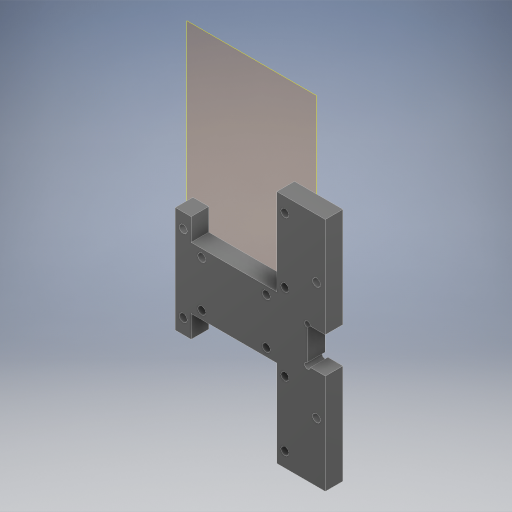
# Autodesk Inventor part: hip joint connector
Saved by Autodesk Inventor 2024 (Build 280153000, 153)
## iProperties
Created: 2024-09-03
Part Number: hip joint connector
Material: PMMA 플라스틱
Document SubType Name: Modeling
Designer: msi
Density: 1.188 g/cm^3
Appearance: 매끄러움 - 검은색
Mass: 12.8648 g
Surface Area: 57.0259 cm^2
Volume: 10.8289 cm^3
Author: msi
Autodesk Inventor part; units mm, degrees
ref_plane "YZ Plane" through (0, 0, 0) normal (1, 0, 0) x (0, 1, 0)
ref_plane "XZ Plane" through (0, 0, 0) normal (0, 1, 0) x (-1, 0, 0)
ref_plane "XY Plane" through (0, 0, 0) normal (0, 0, 1) x (1, 0, 0)
ref_plane "작업 평면1" through (0, 0, 0) normal (0, 0, 1) x (1, 0, 0)
sketch "스케치1" plane through (0, 0, 0) normal (0, 0, 1) x (1, 0, 0)
  arc A0 (-19.5808, 6.2636) -> (-20.1, 4.5766) centre (-17.1, 4.5766) ccw projected
  line L0 (-20.1, -39.6766) -> (-20.1, 4.5766) projected
  arc A1 (-20.1, -39.6766) -> (-19.5808, -41.3636) centre (-17.1, -39.6766) ccw projected
  line L1 (-15.8929, -46.7869) -> (-19.5808, -41.3636) projected
  arc A2 (-15.8929, -46.7869) -> (-13.4121, -48.1) centre (-13.4121, -45.1) ccw projected
  line L2 (13.4121, -48.1) -> (-13.4121, -48.1) projected
  arc A3 (13.4121, -48.1) -> (15.8929, -46.7869) centre (13.4121, -45.1) ccw projected
  line L3 (19.5808, -41.3636) -> (15.8929, -46.7869) projected
  arc A4 (19.5808, -41.3636) -> (20.1, -39.6766) centre (17.1, -39.6766) ccw projected
  line L4 (20.1, 4.5766) -> (20.1, -39.6766) projected
  arc A5 (20.1, 4.5766) -> (19.5808, 6.2636) centre (17.1, 4.5766) ccw projected
  line L5 (15.5953, 12.1246) -> (19.5808, 6.2636) projected
  arc A6 (15.5953, 12.1246) -> (13.9414, 13) centre (13.9414, 11) ccw projected
  line L6 (7.65, 13) -> (13.9414, 13) projected
  arc A7 (9.15, 11.5) -> (7.65, 13) centre (7.65, 11.5) ccw projected
  line L7 (9.15, 11.5) -> (9.15, 10) projected
  arc A8 (9.15, 10) -> (11.5, 7.65) centre (11.5, 10) ccw projected
  line L8 (11.5, 7.65) -> (13.5, 7.65) projected
  arc A9 (14.5, 6.65) -> (13.5, 7.65) centre (13.5, 6.65) ccw projected
  line L9 (14.5, 6.65) -> (14.5, -36.15) projected
  arc A10 (13.5, -37.15) -> (14.5, -36.15) centre (13.5, -36.15) ccw projected
  line L10 (13.5, -37.15) -> (11.5, -37.15) projected
  arc A11 (11.5, -37.15) -> (9.15, -39.5) centre (11.5, -39.5) ccw projected
  line L11 (9.15, -39.5) -> (9.15, -41.5) projected
  arc A12 (8.15, -42.5) -> (9.15, -41.5) centre (8.15, -41.5) ccw projected
  line L12 (8.15, -42.5) -> (-8.15, -42.5) projected
  arc A13 (-9.15, -41.5) -> (-8.15, -42.5) centre (-8.15, -41.5) ccw projected
  line L13 (-9.15, -41.5) -> (-9.15, -39.5) projected
  arc A14 (-9.15, -39.5) -> (-11.5, -37.15) centre (-11.5, -39.5) ccw projected
  line L14 (-11.5, -37.15) -> (-13.5, -37.15) projected
  arc A15 (-14.5, -36.15) -> (-13.5, -37.15) centre (-13.5, -36.15) ccw projected
  line L15 (-14.5, -36.15) -> (-14.5, 6.65) projected
  arc A16 (-13.5, 7.65) -> (-14.5, 6.65) centre (-13.5, 6.65) ccw projected
  line L16 (-13.5, 7.65) -> (-11.5, 7.65) projected
  arc A17 (-11.5, 7.65) -> (-9.15, 10) centre (-11.5, 10) ccw projected
  line L17 (-9.15, 10) -> (-9.15, 11.5) projected
  arc A18 (-7.65, 13) -> (-9.15, 11.5) centre (-7.65, 11.5) ccw projected
  line L18 (-13.9414, 13) -> (-7.65, 13) projected
  arc A19 (-13.9414, 13) -> (-15.5953, 12.1246) centre (-13.9414, 11) ccw projected
  line L19 (-19.5808, 6.2636) -> (-15.5953, 12.1246) projected
  circle A20 centre (17.3, 4) radius 1.35 projected
  circle A21 centre (17.3, -18) radius 1.35 projected
  circle A22 centre (11, -45.3) radius 1.35 projected
  circle A23 centre (-17.3, 4) radius 1.35 projected
  circle A24 centre (-17.3, -18) radius 1.35 projected
  circle A25 centre (-11, -45.3) radius 1.35 projected
  circle A26 centre (17.3, -40) radius 1.35 projected
  circle A27 centre (-17.3, -40) radius 1.35 projected
  arc A28 (19.5808, -112.4636) -> (20.1, -110.7766) centre (17.1, -110.7766) ccw projected
  line L20 (20.1, -66.5234) -> (20.1, -110.7766) projected
  arc A29 (20.1, -66.5234) -> (19.5808, -64.8364) centre (17.1, -66.5234) ccw projected
  line L21 (15.8929, -59.4131) -> (19.5808, -64.8364) projected
  arc A30 (15.8929, -59.4131) -> (13.4121, -58.1) centre (13.4121, -61.1) ccw projected
  line L22 (-13.4121, -58.1) -> (13.4121, -58.1) projected
  arc A31 (-13.4121, -58.1) -> (-15.8929, -59.4131) centre (-13.4121, -61.1) ccw projected
  line L23 (-19.5808, -64.8364) -> (-15.8929, -59.4131) projected
  arc A32 (-19.5808, -64.8364) -> (-20.1, -66.5234) centre (-17.1, -66.5234) ccw projected
  line L24 (-20.1, -110.7766) -> (-20.1, -66.5234) projected
  arc A33 (-20.1, -110.7766) -> (-19.5808, -112.4636) centre (-17.1, -110.7766) ccw projected
  line L25 (-15.5953, -118.3246) -> (-19.5808, -112.4636) projected
  arc A34 (-15.5953, -118.3246) -> (-13.9414, -119.2) centre (-13.9414, -117.2) ccw projected
  line L26 (-7.65, -119.2) -> (-13.9414, -119.2) projected
  arc A35 (-9.15, -117.7) -> (-7.65, -119.2) centre (-7.65, -117.7) ccw projected
  line L27 (-9.15, -117.7) -> (-9.15, -116.2) projected
  arc A36 (-9.15, -116.2) -> (-11.5, -113.85) centre (-11.5, -116.2) ccw projected
  line L28 (-11.5, -113.85) -> (-13.5, -113.85) projected
  arc A37 (-14.5, -112.85) -> (-13.5, -113.85) centre (-13.5, -112.85) ccw projected
  line L29 (-14.5, -112.85) -> (-14.5, -70.05) projected
  arc A38 (-13.5, -69.05) -> (-14.5, -70.05) centre (-13.5, -70.05) ccw projected
  line L30 (-13.5, -69.05) -> (-11.5, -69.05) projected
  arc A39 (-11.5, -69.05) -> (-9.15, -66.7) centre (-11.5, -66.7) ccw projected
  line L31 (-9.15, -66.7) -> (-9.15, -64.7) projected
  arc A40 (-8.15, -63.7) -> (-9.15, -64.7) centre (-8.15, -64.7) ccw projected
  line L32 (-8.15, -63.7) -> (8.15, -63.7) projected
  arc A41 (9.15, -64.7) -> (8.15, -63.7) centre (8.15, -64.7) ccw projected
  line L33 (9.15, -64.7) -> (9.15, -66.7) projected
  arc A42 (9.15, -66.7) -> (11.5, -69.05) centre (11.5, -66.7) ccw projected
  line L34 (11.5, -69.05) -> (13.5, -69.05) projected
  arc A43 (14.5, -70.05) -> (13.5, -69.05) centre (13.5, -70.05) ccw projected
  line L35 (14.5, -70.05) -> (14.5, -112.85) projected
  arc A44 (13.5, -113.85) -> (14.5, -112.85) centre (13.5, -112.85) ccw projected
  line L36 (13.5, -113.85) -> (11.5, -113.85) projected
  arc A45 (11.5, -113.85) -> (9.15, -116.2) centre (11.5, -116.2) ccw projected
  line L37 (9.15, -116.2) -> (9.15, -117.7) projected
  arc A46 (7.65, -119.2) -> (9.15, -117.7) centre (7.65, -117.7) ccw projected
  line L38 (13.9414, -119.2) -> (7.65, -119.2) projected
  arc A47 (13.9414, -119.2) -> (15.5953, -118.3246) centre (13.9414, -117.2) ccw projected
  line L39 (19.5808, -112.4636) -> (15.5953, -118.3246) projected
  circle A48 centre (-17.3, -110.2) radius 1.35 projected
  circle A49 centre (-17.3, -88.2) radius 1.35 projected
  circle A50 centre (-11, -60.9) radius 1.35 projected
  circle A51 centre (17.3, -110.2) radius 1.35 projected
  circle A52 centre (17.3, -88.2) radius 1.35 projected
  circle A53 centre (11, -60.9) radius 1.35 projected
  circle A54 centre (-17.3, -66.2) radius 1.35 projected
  circle A55 centre (17.3, -66.2) radius 1.35 projected
  line L40 (14.6, -36.15) -> (14.6, 6.65)
  arc A56 (14.6, 6.65) -> (13.5, 7.75) centre (13.5, 6.65) ccw
  line L41 (13.5, 7.75) -> (11.5, 7.75)
  arc A57 (9.25, 10) -> (11.5, 7.75) centre (11.5, 10) ccw
  line L42 (9.25, 10) -> (9.25, 11.5)
  arc A58 (9.25, 11.5) -> (8.4246, 12.9) centre (7.65, 11.5) ccw
  line L43 (8.4246, 12.9) -> (13.9414, 12.9)
  arc A59 (15.5126, 12.0684) -> (13.9414, 12.9) centre (13.9414, 11) ccw
  line L44 (15.5126, 12.0684) -> (19.4981, 6.2073)
  arc A60 (20, 4.5766) -> (19.4981, 6.2073) centre (17.1, 4.5766) ccw
  line L45 (20, 4.5766) -> (20, -13)
  arc A61 (14.5, -47.7882) -> (14.6, -47.7455) centre (13.4121, -45.1) ccw
  arc A62 (-14.6, -47.7455) -> (-14.5, -47.7882) centre (-13.4121, -45.1) ccw
  line L46 (-20, -13) -> (-20, 4.5766)
  arc A63 (-19.4981, 6.2073) -> (-20, 4.5766) centre (-17.1, 4.5766) ccw
  line L47 (-19.4981, 6.2073) -> (-15.5126, 12.0684)
  arc A64 (-13.9414, 12.9) -> (-15.5126, 12.0684) centre (-13.9414, 11) ccw
  line L48 (-13.9414, 12.9) -> (-8.4246, 12.9)
  arc A65 (-8.4246, 12.9) -> (-9.25, 11.5) centre (-7.65, 11.5) ccw
  line L49 (-9.25, 11.5) -> (-9.25, 10)
  arc A66 (-11.5, 7.75) -> (-9.25, 10) centre (-11.5, 10) ccw
  line L50 (-11.5, 7.75) -> (-13.5, 7.75)
  arc A67 (-13.5, 7.75) -> (-14.6, 6.65) centre (-13.5, 6.65) ccw
  line L51 (-14.6, 6.65) -> (-14.6, -36.15)
  arc A68 (-14.6, -36.15) -> (-13.5, -37.25) centre (-13.5, -36.15) ccw
  line L52 (-13.5, -37.25) -> (-11.5, -37.25)
  arc A69 (-9.25, -39.5) -> (-11.5, -37.25) centre (-11.5, -39.5) ccw
  line L53 (-9.25, -39.5) -> (-9.25, -41.5)
  arc A70 (-9.25, -41.5) -> (-8.15, -42.6) centre (-8.15, -41.5) ccw
  line L54 (-8.15, -42.6) -> (8.15, -42.6)
  arc A71 (8.15, -42.6) -> (9.25, -41.5) centre (8.15, -41.5) ccw
  line L55 (9.25, -41.5) -> (9.25, -39.5)
  arc A72 (11.5, -37.25) -> (9.25, -39.5) centre (11.5, -39.5) ccw
  line L56 (11.5, -37.25) -> (13.5, -37.25)
  arc A73 (13.5, -37.25) -> (14.6, -36.15) centre (13.5, -36.15) ccw
  line L57 (17.3, -88.2) -> (17.3, -93.2)
  line L58 (17.3, -93.2) -> (20, -93.2)
  line L59 (17.3, -13) -> (20, -13)
  line L60 (17.3, -13) -> (14.6, -13)
  line L61 (17.3, -93.2) -> (14.6, -93.2)
  line L62 (14.6, -13) -> (14.6, -93.2)
  line L63 (20, -13) -> (30, -13)
  line L64 (25, -93.2) -> (20, -93.2)
  circle A74 centre (17.3, -18) radius 1.35
  circle A75 centre (17.3, -40) radius 1.35
  circle A76 centre (17.3, -66.2) radius 1.35
  circle A77 centre (17.3, -88.2) radius 1.35
  line L65 (-14.6, -13) -> (-14.6, -93.2)
  line L66 (14.6, -93.2) -> (14.5, -93.2)
  line L67 (-14.6, -93.2) -> (-20.1, -93.2)
  line L68 (-14.6, -13) -> (-14.5, -13) construction
  line L69 (14.5, -13) -> (65.6, -13) construction
  line L70 (14.6, -13) -> (14.5, -13)
  line L71 (-14.5, -13) -> (-20, -13)
  line L72 (-20, -13) -> (-20.1, -13)
  line L73 (-20.1, -93.2) -> (-20, -93.2)
  circle A78 centre (-17.3, -18) radius 1.35
  circle A79 centre (-17.3, -40) radius 1.35
  circle A80 centre (-17.3, -88.2) radius 1.35
  line L74 (30, -13) -> (35, -13)
  line L75 (35, -13) -> (35, -93.2)
  line L76 (35, -93.2) -> (30, -93.2)
  line L77 (30, -26.0412) -> (30, -25.8633)
  line L78 (30, -25.8633) -> (30, -26.0412)
  line L79 (30, -37.25) -> (30, -37.15)
  line L80 (30, -37.15) -> (30, -37.25)
  line L81 (30, -42.5) -> (30, -42.6)
  line L82 (30, -48) -> (30, -48.1)
  line L83 (35, -47) -> (28.9, -47)
  line L84 (28.9, -59.2) -> (35, -59.2)
  line L85 (35, -59.2) -> (35, -47)
  line L86 (25, -93.2) -> (25, -13)
  line L87 (25, -47) -> (31.1, -47)
  line L88 (31.1, -47) -> (31.1, -59.2)
  line L89 (31.1, -59.2) -> (25, -59.2)
  line L90 (25, -59.2) -> (25, -47)
  line L91 (31.1, -47) -> (31.1, -13)
  line L92 (31.1, -59.2) -> (31.1, -93.2)
  line L93 (25, -93.2) -> (30, -93.2)
  circle A81 centre (28.1, -33.1) radius 1.35
  circle A82 centre (28.1, -73.1) radius 1.35
  line L94 (8.15, -42.6) -> (14.6, -42.6)
  line L95 (8.15, -63.6) -> (-8.15, -63.6)
  arc A83 (-8.15, -63.6) -> (-9.25, -64.7) centre (-8.15, -64.7) ccw
  line L96 (-9.25, -64.7) -> (-9.25, -66.7)
  arc A84 (-11.5, -68.95) -> (-9.25, -66.7) centre (-11.5, -66.7) ccw
  line L97 (-11.5, -68.95) -> (-13.5, -68.95)
  arc A85 (-13.5, -68.95) -> (-14.6, -70.05) centre (-13.5, -70.05) ccw
  line L98 (-14.6, -70.05) -> (-14.6, -112.85)
  arc A86 (-14.6, -112.85) -> (-13.5, -113.95) centre (-13.5, -112.85) ccw
  line L99 (-13.5, -113.95) -> (-11.5, -113.95)
  arc A87 (-9.25, -116.2) -> (-11.5, -113.95) centre (-11.5, -116.2) ccw
  line L100 (-9.25, -116.2) -> (-9.25, -117.7)
  arc A88 (-9.25, -117.7) -> (-8.4246, -119.1) centre (-7.65, -117.7) ccw
  line L101 (-8.4246, -119.1) -> (-13.9414, -119.1)
  arc A89 (-15.5126, -118.2684) -> (-13.9414, -119.1) centre (-13.9414, -117.2) ccw
  line L102 (-15.5126, -118.2684) -> (-19.4981, -112.4073)
  arc A90 (-20, -110.7766) -> (-19.4981, -112.4073) centre (-17.1, -110.7766) ccw
  line L103 (-20, -110.7766) -> (-20, -66.5234)
  arc A91 (15.8102, -59.4693) -> (14.6, -58.4545) centre (13.4121, -61.1) ccw
  line L104 (15.8102, -59.4693) -> (19.4981, -64.8927)
  arc A92 (20, -66.5234) -> (19.4981, -64.8927) centre (17.1, -66.5234) ccw
  line L105 (20, -66.5234) -> (20, -110.7766)
  arc A93 (19.4981, -112.4073) -> (20, -110.7766) centre (17.1, -110.7766) ccw
  line L106 (19.4981, -112.4073) -> (15.5126, -118.2684)
  arc A94 (13.9414, -119.1) -> (15.5126, -118.2684) centre (13.9414, -117.2) ccw
  line L107 (13.9414, -119.1) -> (8.4246, -119.1)
  arc A95 (8.4246, -119.1) -> (9.25, -117.7) centre (7.65, -117.7) ccw
  line L108 (9.25, -117.7) -> (9.25, -116.2)
  arc A96 (11.5, -113.95) -> (9.25, -116.2) centre (11.5, -116.2) ccw
  line L109 (11.5, -113.95) -> (13.5, -113.95)
  arc A97 (13.5, -113.95) -> (14.6, -112.85) centre (13.5, -112.85) ccw
  line L110 (14.6, -112.85) -> (14.6, -70.05)
  arc A98 (14.6, -70.05) -> (13.5, -68.95) centre (13.5, -70.05) ccw
  line L111 (13.5, -68.95) -> (11.5, -68.95)
  arc A99 (9.25, -66.7) -> (11.5, -68.95) centre (11.5, -66.7) ccw
  line L112 (9.25, -66.7) -> (9.25, -64.7)
  arc A100 (9.25, -64.7) -> (8.15, -63.6) centre (8.15, -64.7) ccw
  line L113 (14.6, -42.6) -> (-9.25, -42.6)
  line L114 (-9.25, -63.6) -> (14.6, -63.6)
  line L115 (14.6, -63.6) -> (14.6, -42.6)
  circle A101 centre (11, -45.3) radius 1.35
  circle A102 centre (11, -60.9) radius 1.35
  circle A103 centre (-11, -45.3) radius 1.35
  circle A104 centre (-11, -60.9) radius 1.35
  line L116 (-9.25, -42.6) -> (-14.6, -42.6)
  line L117 (-14.6, -42.6) -> (-14.6, -63.6)
  line L118 (-14.6, -63.6) -> (-9.25, -63.6)
  line L119 (-20, -13) -> (-20, -93.2)
  circle A105 centre (-17.3, -66.2) radius 1.35
  line L120 (-20, -35) -> (-14.6, -35)
  line L121 (-17.3, -71.2) -> (-14.6, -71.2)
  line L122 (-17.3, -71.2) -> (-20, -71.2)
  point P0 (0, 0)
  point P1 (30, -93.2)
  point P2 (25, -13)
  point P3 (-8.15, -42.6)
  point P4 (-14.6, -42.6)
  dimension "d0" = 0.1
  dimension "d2" = 5
  dimension "d3" = 5
  dimension "d4" = 5
  dimension "d5" = 2.7
  dimension "d6" = 2.7
  dimension "d7" = 2.7
  dimension "d8" = 2.7
  dimension "d11" = 2.7
  dimension "d12" = 2.7
  dimension "d14" = 2.7
  dimension "d16" = 6.1
  dimension "d17" = 12.2
  dimension "d31" = 6.1
  dimension "d36" = 2.7
  dimension "d37" = 2.7
  dimension "d40" = 0.1
  dimension "d41" = 2.7
  dimension "d42" = 2.7
  dimension "d43" = 2.7
  dimension "d44" = 2.7
  constraints: 166 end point, 73 point on circle, 50 centre point, 35 point on line, 16 perpendicular, 12 coincident, 11 horizontal, 10 parallel, 2 vertical, 1 collinear, 1 concentric, 1 tangent, 62 other
  measures "d0" distance between parallel lines of L9 L40
  measures "d2" distance of L57.start L57.end
  measures "d3" distance of A21.centre L59.start
  measures "d4" distance of L64.start L64.end
  measures "d5" diameter of A74
  measures "d6" diameter of A75
  measures "d7" diameter of A76
  measures "d8" diameter of A77
  measures "d11" diameter of A78
  measures "d12" diameter of A79
  measures "d14" diameter of A80
  measures "d16" distance of L84.end L84.start
  measures "d17" distance of L84.start L83.end
  measures "d31" distance of L88.end L89.end
  measures "d36" diameter of A81
  measures "d37" diameter of A82
  measures "d40" distance between parallel lines of L32 L95
  measures "d41" diameter of A101
  measures "d42" diameter of A102
  measures "d43" diameter of A103
  measures "d44" diameter of A104
extrude "돌출5" add sketch "스케치1" along normal blind 6 contours L119 L120 L51 L65 A2 L1 A1 | A1 L1 A2 L65 A31 L23 A32 L119 | A32 L23 A31 L65 L121 L122 L103 L119 | L65 L116 L113 L54 L94 L62 A3 L2 A2 | A2 L2 A3 L62 A30 L22 A31 L65 | A31 L22 A30 L62 L114 L95 L118 L65 | L62 L40 L60 L59 L63 L4 A4 L3 A3 | A3 L3 A4 L4 L63 L86 L64 L20 A29 L21 A30 L62 | A30 L21 A29 L20 L64 L105 A92 L104 A91 L62 | A91 L104 A92 L105 L58 L61 L62 | L63 L74 L91 L83 L87 L86 | L86 L89 L84 L92 L76 L93
sketch "스케치2" plane through (0, 0, 6) normal (0, 0, 1) x (1, 0, 0)
  line L0 (25, -47) -> (31.1, -47) projected
  line L1 (25, -59.2) -> (25, -47) projected
  line L2 (31.1, -59.2) -> (25, -59.2) projected
  circle A0 centre (25, -47) radius 1
  circle A1 centre (25, -59.2) radius 1
  point P0 (0, 0)
  dimension "d49" = 2
  dimension "d50" = 2
  constraints: 2 centre point, 2 coincident
  measures "d49" diameter of A0
  measures "d50" diameter of A1
extrude "돌출6" cut sketch "스케치2" against normal blind 6
